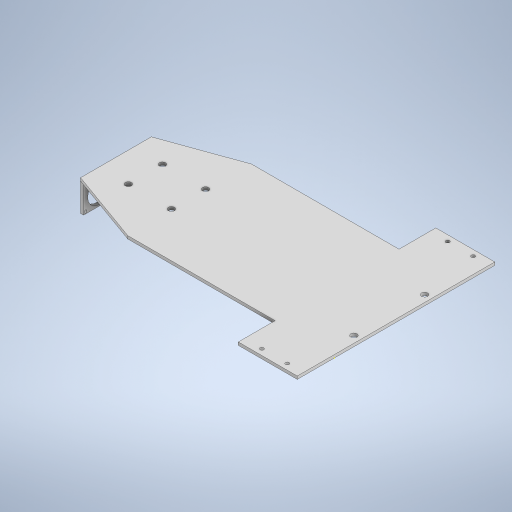
# Autodesk Inventor part: robocik
Saved by Autodesk Inventor 2024.2 (Build 282272000, 272)
## iProperties
Created: 2024-04-19
Part Number: robocik
Material: Ogólny
Document SubType Name: Modeling
Designer: rjane
Density: 1 g/cm^3
Appearance: Domyślna
Author: rjane
Autodesk Inventor part; units mm, degrees
ref_plane "YZ Plane" through (0, 0, 0) normal (1, 0, 0) x (0, 1, 0)
ref_plane "XZ Plane" through (0, 0, 0) normal (0, 1, 0) x (-1, 0, 0)
ref_plane "XY Plane" through (0, 0, 0) normal (0, 0, 1) x (1, 0, 0)
sketch "Szkic1" plane through (0, 0, 0) normal (0, 1, 0) x (-1, 0, 0)
  point P0 (0, 0)
sketch "Szkic2" plane through (0, 0, 0) normal (0, 1, 0) x (-1, 0, 0)
  line L0 (0, 0) -> (140, 0)
  line L1 (190, -18) -> (190, -66)
  line L2 (140, -84) -> (0, -84)
  line L3 (0, -84) -> (0, 0)
  line L4 (140, 0) -> (190, -18)
  line L5 (190, -66) -> (140, -84)
  circle A0 centre (170, -30.4) radius 2.1
  circle A1 centre (170, -53.6) radius 2.1
  line L6 (190, -42) -> (110.3864, -42)
  circle A2 centre (140.8, -30.4) radius 2.1
  circle A3 centre (140.8, -53.6) radius 2.1
  circle A4 centre (10.75, 21) radius 1.25
  circle A5 centre (10.75, -105) radius 1.25
  circle A6 centre (28, 21) radius 1.25
  circle A7 centre (28, -105) radius 1.25
  line L7 (0, -84) -> (40, -84)
  line L8 (40, -84) -> (40, -109)
  line L9 (40, -109) -> (0, -109)
  line L10 (0, -109) -> (0, -84)
  line L11 (0, 0) -> (40, 0)
  line L12 (40, 0) -> (40, 25)
  line L13 (40, 25) -> (0, 25)
  line L14 (0, 25) -> (0, 0)
  circle A8 centre (4.5993, -66) radius 2.1
  circle A9 centre (4.5993, -18) radius 2.1
  point P0 (20, -84)
  point P1 (20, -109)
  point P2 (40, -96.5)
  point P3 (40, 12.5)
  point P4 (0, 12.5)
  point P5 (40, 0)
  point P6 (40, -84)
  dimension "d3" = 48
  dimension "d4" = 140
  dimension "d5" = 84
  dimension "d6" = 4.2
  dimension "d7" = 4.2
  dimension "d8" = 23.2
  dimension "d9" = 11.6
  dimension "d10" = 4.2
  dimension "d11" = 29.2
  dimension "d12" = 4.2
  dimension "d13" = 2.5
  dimension "d14" = 2.5
  dimension "d15" = 2.5
  dimension "d16" = 2.5
  dimension "d17" = 28
  dimension "d18" = 28
  dimension "d19" = 42
  dimension "d20" = 50
  dimension "d21" = 50
  dimension "d46" = 17.25
  dimension "d47" = 17.25
  dimension "d73" = 23.2
  dimension "d74" = 29.2
  dimension "d78" = 20
  dimension "d79" = 20
  dimension "d80" = 49.2
  dimension "d83" = 25
  dimension "d84" = 40
  dimension "d85" = 25
  dimension "d86" = 40
  dimension "d87" = 4
  dimension "d88" = 4
  dimension "d89" = 4
  dimension "d90" = 4
  dimension "d91" = 4.2
  dimension "d92" = 4.2
  dimension "d93" = 18
  dimension "d94" = 18
  constraints: 30 end point, 10 centre point, 6 midpoint, 6 parallel, 3 horizontal, 3 perpendicular
  measures "d3" distance of L1.start L1.end
  measures "d4" distance of L0.start L0.end
  measures "d5" distance of L2.end L0.start
  measures "d6" diameter of A0
  measures "d7" diameter of A1
  measures "d8" distance of A1.centre A0.centre
  measures "d9" distance from line of L6 A0.centre
  measures "d10" diameter of A2
  measures "d11" distance of A0.centre A2.centre
  measures "d12" diameter of A3
  measures "d13" diameter of A4
  measures "d14" diameter of A5
  measures "d15" diameter of A6
  measures "d16" diameter of A7
  measures "d17" distance from line of L3 A6.centre
  measures "d18" distance from line of L3 A7.centre
  measures "d19" distance between parallel lines of L0 L6
  measures "d20" horizontal distance of L1.end L2.start
  measures "d21" horizontal distance of L0.end L1.start
  measures "d46" distance of A4.centre A6.centre
  measures "d47" distance of A5.centre A7.centre
  measures "d73" distance of A3.centre A2.centre
  measures "d74" distance of A3.centre A1.centre
  measures "d78" distance from line of L1 A1.centre
  measures "d79" distance from line of L1 A0.centre
  measures "d80" distance from line of L1 A3.centre
  measures "d83" distance of point (20, -84) point (20, -109)
  measures "d84" distance from line of point (40, -96.5) L10
  measures "d85" distance between parallel lines of L13 L11
  measures "d86" distance of point (40, 12.5) point (0, 12.5)
  measures "d87" distance from line of L13 A4.centre
  measures "d88" distance from line of L13 A6.centre
  measures "d89" distance from line of L9 A7.centre
  measures "d90" distance from line of L9 A5.centre
  measures "d91" diameter of A8
  measures "d92" diameter of A9
  measures "d93" distance from line of L7 A8.centre
  measures "d94" distance from line of L0 A9.centre
extrude "Wyciągnięcie proste1" add sketch "Szkic2" along normal blind 2
sketch "Szkic3" plane through (-190, 0, -66) normal (-1, 0, 0) x (0, 0, 1)
  line L0 (0, 2) -> (48, 2) projected
  line L1 (48, 2) -> (0, 2)
  line L2 (0, 2) -> (0, -19)
  line L3 (0, -19) -> (48, -19)
  line L4 (48, -19) -> (48, 2)
  circle A0 centre (37.195, -10) radius 8
  line L5 (0, 0) -> (48, 0) projected
  circle A1 centre (10.805, -10) radius 8
  circle A2 centre (46.6, -1.4) radius 1
  circle A3 centre (46.6, -17.6) radius 1
  circle A4 centre (1.4, -17.6) radius 1
  circle A5 centre (1.4, -1.4) radius 1
  point P0 (66, 0)
  dimension "d24" = 48
  dimension "d25" = 21
  dimension "d26" = 10
  dimension "d28" = 16
  dimension "d29" = 10
  dimension "d31" = 16
  dimension "d32" = 1.4
  dimension "d33" = 1.4
  dimension "d34" = 1.4
  dimension "d35" = 1.4
  dimension "d36" = 1.4
  dimension "d37" = 1.4
  dimension "d38" = 1.4
  dimension "d39" = 1.4
  dimension "d40" = 2
  dimension "d41" = 2
  dimension "d42" = 2
  dimension "d43" = 2
  dimension "d75" = 26.39
  dimension "d76" = 10.805
  dimension "d77" = 10.805
  constraints: 8 end point, 6 centre point, 2 parallel, 1 horizontal, 1 perpendicular
  measures "d24" distance of L2.end L3.end
  measures "d25" distance of L1.end L2.end
  measures "d26" distance from line of L5 A0.centre
  measures "d28" diameter of A0
  measures "d29" distance from line of L5 A1.centre
  measures "d31" diameter of A1
  measures "d32" distance from line of L4 A2.centre
  measures "d33" distance from line of L5 A2.centre
  measures "d34" distance from line of L3 A3.centre
  measures "d35" distance from line of L4 A3.centre
  measures "d36" distance from line of L2 A4.centre
  measures "d37" distance from line of L3 A4.centre
  measures "d38" distance from line of L2 A5.centre
  measures "d39" distance from line of L5 A5.centre
  measures "d40" diameter of A3
  measures "d41" diameter of A2
  measures "d42" diameter of A4
  measures "d43" diameter of A5
  measures "d75" distance of A1.centre A0.centre
  measures "d76" distance from line of L4 A0.centre
  measures "d77" distance from line of L2 A1.centre
extrude "Wyciągnięcie proste2" add sketch "Szkic3" against normal blind 2 contours L5 L4 L3 L2
sketch "Szkic4" plane through (0, 0, 0) normal (0, -1, 0) x (1, 0, 0)
  line L0 (-140, 0) -> (0, 0) projected
  line L1 (-40, -84) -> (-140, -84) projected
  line L2 (-55, -84) -> (-55, 0)
  line L3 (0, 0) -> (0, -109) projected
  line L4 (-125, -84) -> (-125, 0)
  circle A0 centre (-65.9, -29.27) radius 1.375
  circle A1 centre (-114.07, -28) radius 1.375
  circle A2 centre (-81.25, -79.81) radius 1.375
  point P0 (0, -84)
  point P1 (-70, 0)
  dimension "d60" = 55
  dimension "d61" = 70
  dimension "d62" = 2.75
  dimension "d63" = 10.9
  dimension "d64" = 29.27
  dimension "d65" = 2.75
  dimension "d66" = 28
  dimension "d67" = 59.07
  dimension "d68" = 79.81
  dimension "d69" = 2.75
  dimension "d70" = 26.25
  constraints: 4 end point, 4 point on line, 3 centre point, 2 perpendicular, 1 midpoint
  measures "d60" distance between parallel lines of L2 L3
  measures "d61" distance between parallel lines of L4 L2
  measures "d62" diameter of A0
  measures "d63" distance from line of L2 A0.centre
  measures "d64" distance from line of L0 A0.centre
  measures "d65" diameter of A1
  measures "d66" distance from line of L0 A1.centre
  measures "d67" distance from line of L2 A1.centre
  measures "d68" vertical distance of point (-70, 0) A2.centre
  measures "d69" diameter of A2
  measures "d70" distance from line of L2 A2.centre
extrude "Wyciągnięcie proste3" add sketch "Szkic4" along normal blind 16 contours A0 | A1 | A2
